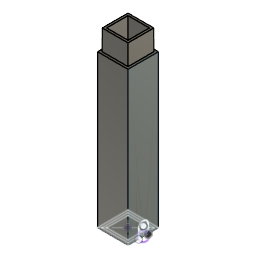
tower (Autodesk Fusion 360 design; units mm, degrees)
Autodesk Fusion 360 part; units mm, degrees
sketch "Sketch1" plane through (0, 0, 0) normal (0, 0, 1) x (1, 0, 0)
  line L0 (20, -20) -> (-20, -20)
  line L1 (-20, -20) -> (-20, 20)
  line L2 (-20, 20) -> (20, 20)
  line L3 (20, 20) -> (20, -20)
  line L4 (20, -20) -> (-20, 20) construction
  line L5 (-20, -20) -> (20, 20) construction
  line L6 (-17, -17) -> (-17, 17)
  line L7 (-17, 17) -> (17, 17)
  line L8 (17, 17) -> (17, -17)
  line L9 (17, -17) -> (-17, -17)
  line L10 (-14, -14) -> (-14, 14)
  line L11 (-14, 14) -> (14, 14)
  line L12 (14, 14) -> (14, -14)
  line L13 (14, -14) -> (-14, -14)
  dimension "d1" = 40
  dimension "d2" = 40
  dimension "d3" = 3
  dimension "d4" = 6
  constraint horizontal L0
  constraint perpendicular L0 L1
  constraint parallel L0 L2
  constraint parallel L1 L3
  constraint coincident L4 origin
  constraint coincident L5 origin
  measures "d1" distance of L1.end L2.end
  measures "d2" distance of L0.end L1.end
extrude "Extrude1" add sketch "Sketch1" along normal blind 200 contours L0 L1 L2 L3 makes body 1
extrude "Extrude2" add sketch "Sketch1" along normal blind 27 draft -0.1 from surface at 200 separate body contours L6 L7 L8 L9 makes body 2
extrude "Extrude3" add 1 faces at (4.6667, -16, 200) along direction (0, 0, -1) blind 20 on bodies 2 bodies 1 2
chamfer "Chamfer1" distance 3 angle 45 4 edges at (0, 14, 180) (-14, 0, 180) (0, -14, 180) (14, 0, 180) on bodies 1
extrude "Extrude4" add sketch "Sketch1" along normal blind 2 contours L6 L7 L8 L9 | L10 L11 L12 L13 bodies 1
sketch "Sketch2" plane through (20, 0, 0) normal (1, 0, 0) x (0, 1, 0)
  line L0 (-20, 0) -> (20, 0)
  line L1 (20, 0) -> (20, 200)
  line L2 (20, 200) -> (-20, 200)
  line L3 (-20, 200) -> (-20, 0)
  circle A0 centre (0, 12) radius 4
  circle A1 centre (0, 12) radius 6
  line L4 (-6, 12) -> (-6, -0.3727)
  line L5 (6, 12) -> (6, 0)
  dimension "d15" = 8
  dimension "d16" = 12
  dimension "d17" = 2
  constraint vertical A0.centre origin
  constraint coincident A1 L4.start
  constraint perpendicular L0 L4
  constraint coincident A1 L5.start
  constraint coincident L0 L5.end
  constraint perpendicular L0 L5
  constraint tangent A1 L5
  constraint tangent A1 L4
  measures "d15" diameter of A0
  measures "d16" distance of A0.centre origin
extrude "Extrude5" add sketch "Sketch2" against normal blind 7 contours L0 A1 L4 L5 | A1 | A0 bodies 1
mirror "Mirror1" about plane through (0, 0, 0) normal (1, 0, 0) of "Extrude5"
hole "Hole1" at (20, 0, 12) direction (-1, 0, 0) diameter 8 end up to surface (40 mm away) bodies 1
